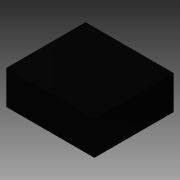
# Autodesk Inventor part: 10UH
Saved by Autodesk Inventor 2015 SP1 (Build 190203100, 203)
## iProperties
Created: 2015-10-19
Part Number: 10UH
Material: Generic
Document SubType Name: Modeling
Designer: Kartikye
Density: 1 g/cm^3
Appearance: IND_ELL6XH, 10UH
Author: Kartikye
Autodesk Inventor part; units mm, degrees
ref_plane "YZ Plane" through (0, 0, 0) normal (1, 0, 0) x (0, 1, 0)
ref_plane "XZ Plane" through (0, 0, 0) normal (0, 1, 0) x (-1, 0, 0)
ref_plane "XY Plane" through (0, 0, 0) normal (0, 0, 1) x (1, 0, 0)
sketch "IND_ELL6XH, 10UH_40" plane through (0, 0, 0) normal (0, 0, 1) x (1, 0, 0)
  line L0 (-3.937, 3.5052) -> (3.937, 3.5052)
  line L1 (3.937, 3.5052) -> (3.937, -3.5814)
  line L2 (3.937, -3.5814) -> (-3.937, -3.5814)
  line L3 (-3.937, -3.5814) -> (-3.937, 3.5052)
  constraints: 8 end point
extrude "Extrusion1" add sketch "IND_ELL6XH, 10UH_40" along normal blind 3
body "Solid1"
